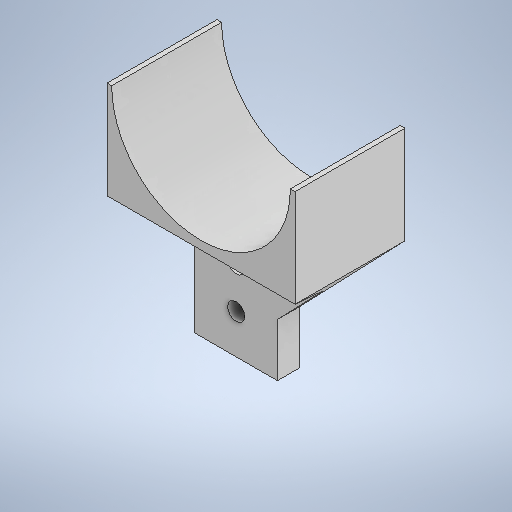
# Autodesk Inventor part: motorsupport
Saved by Autodesk Inventor 2025.2 (Build 292293000, 293)
## iProperties
Created: 2025-01-03
Part Number: motorsupport
Material: Generic
Document SubType Name: Modeling
Designer: email
Density: 1 g/cm^3
Appearance: Default
Author: email
Autodesk Inventor part; units mm, degrees
ref_plane "YZ Plane" through (0, 0, 0) normal (1, 0, 0) x (0, 1, 0)
ref_plane "XZ Plane" through (0, 0, 0) normal (0, 1, 0) x (-1, 0, 0)
ref_plane "XY Plane" through (0, 0, 0) normal (0, 0, 1) x (1, 0, 0)
sketch "Sketch1" plane through (0, 0, 0) normal (0, 0, 1) x (1, 0, 0)
  line L0 (0, 0) -> (30, 0)
  line L1 (30, 0) -> (30, 40)
  line L2 (30, 40) -> (0, 40)
  line L3 (0, 40) -> (0, 0)
  circle A0 centre (15, 10) radius 3.125
  circle A1 centre (15, -5) radius 3.125
  line L4 (51.875, 74) -> (51.875, 6) construction
  line L5 (51.875, 6) -> (16.525, 6) construction
  line L6 (16.525, 6) -> (16.525, 74)
  line L7 (51.875, 40) -> (34.2, 40)
  line L8 (34.2, 40) -> (34.2, 75.5)
  circle A2 centre (34.2, 75.5) radius 32.5
  line L9 (0, 40) -> (68.4124, 40)
  line L10 (68.4124, 40) -> (68.4124, 75.5)
  line L11 (68.4124, 75.5) -> (0, 75.5)
  line L12 (0, 75.5) -> (0, 40)
  line L13 (68.4124, 40) -> (30, 0)
  line L14 (0, 40) -> (30, 40)
  line L15 (30, 40) -> (30, -19.2784)
  line L16 (30, -19.2784) -> (0, -19.2784)
  line L17 (0, -19.2784) -> (0, 40)
  point P0 (15, 40)
  point P1 (34.2062, 75.5)
  point P2 (1.7, 75.5)
  point P3 (66.7, 75.5)
  dimension "d0" = 30
  dimension "d1" = 15
  dimension "d2" = 15
  dimension "d3" = 40
  dimension "d4" = 6.25
  dimension "d5" = 6.25
  dimension "d6" = 30
  dimension "d7" = 35.35
  dimension "d8" = 13.475
  dimension "d10" = 34
  dimension "d11" = 35.5
  dimension "d12" = 65
  dimension "d13" = 34.2062
  dimension "d15" = 34.2062
  constraints: 36 end point, 7 parallel, 4 horizontal, 4 perpendicular, 3 centre point, 3 midpoint, 1 coincident
  measures "d0" distance of L1.end L2.end
  measures "d1" distance of A1.centre A0.centre
  measures "d2" distance from line of L3 A0.centre
  measures "d3" distance of L0.end L1.end
  measures "d4" diameter of A0
  measures "d5" diameter of A1
  measures "d6" distance of point (15, 40) A0.centre
  measures "d7" distance between parallel lines of L4 L6
  measures "d8" distance between parallel lines of L1 L6
  measures "d10" distance between parallel lines of L2 L5
  measures "d11" distance of L7.end L8.end
  measures "d12" diameter of A2
  measures "d13" distance from line of L12 point (34.206, 75.5)
  measures "d15" distance from line of point (34.206, 75.5) L10
extrude "Extrusion1" add sketch "Sketch1" along normal blind 8 contours L3 L2 L1 L0 | L0 L15 L16 L17 | L1 L9 L7 L13 | L12 L11 A2 L6 L2 | L2 L6 A2 L8 L9 | L9 L7 L8 A2 L11 L10
extrude "Extrusion2" add sketch "Sketch1" along normal blind 40 contours L12 L11 A2 L6 L2 | L2 L6 A2 L8 L9 | L9 L7 L8 A2 L11 L10
chamfer "Chamfer1" distance 32 angle 35 1 edges at (34.2062, 40, 8) measured on face at (22.8041, 40, 18.6667)
body "Solid1"
